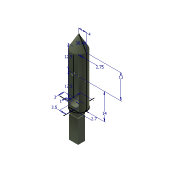
# Autodesk Inventor part: Rotator Frame_xw
Saved by Autodesk Inventor 2016 (Build 200138000, 138)
## iProperties
Created: 2014-06-20
Part Number: Rotator Frame_xw
Document SubType Name: Modeling
Designer: 121767
Density: 1.068 g/cm^3
Material: SAN Plastic
Appearance: Precast Smooth
Author: 121767
Autodesk Inventor part; units mm, degrees
ref_plane "YZ Plane" through (0, 0, 0) normal (1, 0, 0) x (0, 1, 0)
ref_plane "XZ Plane" through (0, 0, 0) normal (0, 1, 0) x (-1, 0, 0)
sketch "Sketch1" plane through (0, 0, 0) normal (0, 0, 1) x (1, 0, 0)
  line L0 (0, 19.9282) -> (4, 13)
  line L1 (4, 13) -> (4, -14)
  line L2 (4, -14) -> (0, -14)
  line L3 (0, -25.9015) -> (0, 19.9282)
  line L4 (2.75, -12.5) -> (-2.75, -12.5)
  line L5 (-2.75, -12.5) -> (-2.75, 12.5)
  line L6 (-2.75, 12.5) -> (2.75, 12.5)
  line L7 (2.75, 12.5) -> (2.75, -12.5)
  point P0 (0, 0)
  dimension "d0" = 30
  dimension "d1" = 4
  dimension "d45" = 14
  dimension "d47" = 2.75
  dimension "d48" = 13
  dimension "d81" = 12.5
  dimension "d82" = 12.5
  constraints: 16 end point, 2 parallel, 2 perpendicular, 1 horizontal, 1 point on line, 1 vertical, 1 other
  measures "d0" angle of L3 L0
  measures "d1" distance between parallel lines of L1 L3
  measures "d45" distance from line of L2 point (0, 0)
  measures "d47" distance between parallel lines of L7 L3
  measures "d48" vertical distance of point (0, 0) L0.end
  measures "d81" distance from line of L6 point (0, 0)
  measures "d82" distance from line of L4 point (0, 0)
revolve "main cylinder" add sketch "Sketch1" angle 360 about axis through (0, -25.9015, 0) along (0, 1, 0) contours L0 L1 L2 L3 L4 L7 L6 | L6 L7 L4 L3
extrude "main window" cut sketch "Sketch1" against normal mid plane 25.4 contours L6 L7 L4 L3 | L3 L4 L5 L6
sketch "Sketch2" plane through (-2.75, -12.5, 2.9047) normal (1, 0, 0) x (0, 0, -1)
  point P0 (2.9047, 12.5)
  point P1 (2.9047, 12.5)
  constraints: 1 coincident
hole "full side hole" at (-2.75, 0, 0) direction (-1, 0, 0) diameter 1 depth 25.4
sketch "Sketch3" plane through (0, -14, 0) normal (0, -1, 0) x (1, 0, 0)
  circle A0 centre (0, 0) radius 4
  line L0 (-3.9686, 0.5) -> (-3.5, 0.5)
  line L1 (-3.5, 0.5) -> (-3.5, -0.5)
  line L2 (-3.5, -0.5) -> (-3.9686, -0.5)
  line L3 (-10.1288, 0) -> (5.4225, 0)
  line L4 (0, 8.0973) -> (0, -8.0973)
  line L5 (-2.9513, 2.7) -> (2.9513, 2.7)
  line L6 (3.9686, 0.5) -> (3.5, 0.5)
  line L7 (3.5, 0.5) -> (3.5, -0.5)
  line L8 (3.5, -0.5) -> (3.9686, -0.5)
  line L9 (-1.75, 2.7) -> (-1.7428, 2.7) construction
  line L10 (1.7428, 1.7526) -> (1.75, 1.7526)
  line L11 (-1.7428, 1.7526) -> (-1.75, 1.7526)
  line L12 (1.7428, 2.7) -> (1.75, 2.7) construction
  line L13 (-1.7428, 2.7) -> (1.7428, 2.7)
  point P0 (0, 0)
  point P1 (0, -3)
  point P2 (0, -7)
  point P3 (-3.5536, -1.8362)
  point P4 (3.5536, -1.8362)
  dimension "d14" = 1
  dimension "d15" = 3.5
  dimension "d20" = 3
  dimension "d35" = 2.7
  dimension "d38" = 7
  constraints: 28 end point, 4 point on line, 2 midpoint, 10 other
  measures "d14" distance between parallel lines of L2 L0
  measures "d15" distance from line of point (0, 0) L1
  measures "d20" distance from line of L3 point (0, -3)
  measures "d35" distance between parallel lines of L3 L5
  measures "d38" distance from line of point (0, -7) L3
hole "partial side hole" at (-2.75, 0, 0) direction (-1, 0, 0) diameter 2 depth 0.75
extrude "side channels" cut sketch "Sketch3" against normal blind 14.5 contours L3 L7 L6 A0 | A0 L8 L7 L3 | A0 L3 L1 L2 | L3 A0 L0 L1
hole "thread hole" at (0, -14, -3) direction (0, 1, 0) diameter 1 end through all
extrude "Extrusion4" cut sketch "Sketch3" against normal blind 10 contours L5 L4 A0 | L4 L5 A0
extrude "Extrusion5" cut sketch "Sketch3" along normal blind 20 contours A0 L3 L1 L2 | L3 A0 L0 L1
fillet "Fillet1" radius 2 4 edges at (-2.75, 12.5, 0) (2.75, 12.5, 0) (-2.75, -12.5, -0.1024) (2.75, -12.5, -0.1024)
mirror "Mirror4" about plane through (0, 0, 0) normal (1, 0, 0) of "partial side hole", "full side hole"
sketch "Sketch8" plane through (0, -14, 0) normal (0, -1, 0) x (1, 0, 0)
  line L0 (2.9513, 2.7) -> (-2.9513, 2.7) projected
  line L1 (2.9513, 2.7) -> (-2.9513, 2.7) projected
  arc A0 (-2.9513, 2.7) -> (-3.9686, 0.5) centre (0, 0) ccw projected
  line L2 (-3.9686, 0.5) -> (-3.5, 0.5) projected
  line L3 (-3.5, 0.5) -> (-3.5, -0.5) projected
  line L4 (-3.5, -0.5) -> (-3.9686, -0.5) projected
  arc A1 (-3.9686, -0.5) -> (3.9686, -0.5) centre (0, 0) ccw projected
  line L5 (3.9686, -0.5) -> (3.5, -0.5) projected
  line L6 (3.5, -0.5) -> (3.5, 0.5) projected
  line L7 (3.5, 0.5) -> (3.9686, 0.5) projected
  arc A2 (3.9686, 0.5) -> (2.9513, 2.7) centre (0, 0) ccw projected
  circle A3 centre (0, -3) radius 0.5 projected
  line L8 (-2.9513, 2.7) -> (2.9513, 2.7) projected
  circle A4 centre (0, 0) radius 4 projected
  line L9 (-2.4, -1) -> (-2.4, 2.7)
  line L10 (2.4, -1) -> (2.4, 2.7)
  line L11 (-2.4, -1) -> (2.4, -1)
  point P0 (0, 15.9155)
  point P1 (0, -1)
  dimension "d105" = 4.8
  dimension "d115" = 1
  constraints: 6 end point, 2 point on line, 1 horizontal, 1 midpoint, 1 perpendicular, 1 vertical, 1 vertical alignment, 1 other
  measures "d105" distance between parallel lines of L10 L9
  measures "d115" distance from line of A0.centre L11
extrude "Extrusion11" add sketch "Sketch8" along normal blind 15 contours L10 L11 L9 L0
ref_plane "Work Plane5" through (0, -16.5, 0) normal (0, -1, 0) x (1, 0, 0)
sketch "Sketch9" plane through (0, -16.5, 0) normal (0, -1, 0) x (1, 0, 0)
  line L0 (2.4, -1) -> (-2.4, -1) projected
  line L1 (-2.4, -1) -> (-2.4, 2.7) projected
  line L2 (2.4, 2.7) -> (2.4, -1) projected
  line L3 (-2.9513, 2.7) -> (2.9513, 2.7) projected
  line L4 (2, 2.5) -> (-2, 2.5)
  line L5 (-2, 2.5) -> (-2, -0.8)
  line L6 (-2, -0.8) -> (2, -0.8)
  line L7 (2, -0.8) -> (2, 2.5)
  point P0 (0, 0)
  point P1 (0, 2.5)
  point P2 (0, -1)
  point P3 (0, -1)
  dimension "d108" = 4
  dimension "d109" = 3.3
  dimension "d111" = 0.2
  dimension "d112" = 0.4
  constraints: 8 end point, 3 midpoint, 2 parallel, 1 coincident, 1 horizontal, 1 perpendicular
  measures "d108" distance of L5.end L6.end
  measures "d109" distance of L6.end L4.start
  measures "d111" distance between parallel lines of L0 L6
  measures "d112" distance between parallel lines of L2 L7
extrude "Extrusion12" cut sketch "Sketch9" along normal blind 0.5
body "Solid1"
